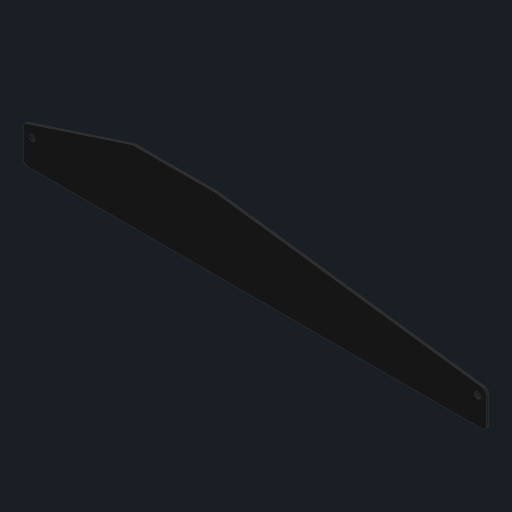
# Autodesk Inventor part: panel
Saved by Autodesk Inventor 2023 (Build 270158000, 158)
## iProperties
Created: 2023-05-11
Part Number: panel
Material: Generic
Document SubType Name: Modeling
Designer: reima
Density: 1 g/cm^3
Appearance: Default
Author: reima
Autodesk Inventor part; units mm, degrees
ref_plane "YZ Plane" through (0, 0, 0) normal (1, 0, 0) x (0, 1, 0)
ref_plane "XZ Plane" through (0, 0, 0) normal (0, 1, 0) x (-1, 0, 0)
ref_plane "XY Plane" through (0, 0, 0) normal (0, 0, 1) x (1, 0, 0)
sketch "Sketch1" plane through (0, 0, 0) normal (0, 0, 1) x (1, 0, 0)
  circle A0 centre (-120.15, 28.2703) radius 2.3114 projected
  circle A1 centre (-437.65, 28.2703) radius 2.3114 projected
  line L0 (-124.0119, 9.2203) -> (-113.8, 9.2203) projected
  line L1 (-113.8, 24.2317) -> (-113.8, 32.2073) projected
  line L2 (-443.67, 33.8077) -> (-443.67, 0.5333) projected
  line L3 (-382.9881, 34.6203) -> (-441.5119, 34.6203) projected
  line L4 (-443.67, 34.6203) -> (-113.8, 34.6203)
  line L5 (-113.8, 31.8362) -> (-113.8, 12.3953)
  line L6 (-116.975, 9.2203) -> (-440.495, 9.2203)
  line L7 (-443.67, 12.3953) -> (-443.67, 32.316)
  arc A2 (-116.975, 9.2203) -> (-113.8, 12.3953) centre (-116.975, 12.3953) ccw
  circle A3 centre (-361.45, 54.8387) radius 2.3114 projected
  line L8 (-306.586, 60.0203) -> (-365.773, 60.0203) projected
  line L9 (-365.773, 60.0203) -> (-441.4793, 35.3346)
  line L10 (-306.586, 60.0203) -> (-116.5603, 34.984)
  arc A4 (-443.67, 12.3953) -> (-440.495, 9.2203) centre (-440.495, 12.3953) ccw
  arc A5 (-441.4793, 35.3346) -> (-443.67, 32.316) centre (-440.495, 32.316) ccw
  arc A6 (-113.8, 31.8362) -> (-116.5603, 34.984) centre (-116.975, 31.8362) ccw
  line L11 (-306.586, 60.0203) -> (-365.773, 60.0203)
  point P0 (0, 0)
  dimension "d0" = 3.175
  dimension "d1" = 3.175
  constraints: 14 end point, 8 point on circle, 8 tangent, 7 point on line, 4 centre point, 2 equal radius, 2 parallel, 1 collinear, 1 horizontal, 1 perpendicular
  measures "d0" radius of A2
  measures "d1" radius of A4
extrude "Extrusion1" add sketch "Sketch1" along normal blind 1.5875
sketch "Sketch2" plane through (0, 0, 1.5875) normal (0, 0, 1) x (1, 0, 0)
  circle A0 centre (-361.45, 54.8387) radius 2.3114 projected
  circle A1 centre (-361.45, 54.8387) radius 2.3114
  point P0 (0, 0)
  constraints: 1 centre point, 1 coincident
extrude "Extrusion2" add sketch "Sketch2" against normal blind 1.5875
body "Solid1"
